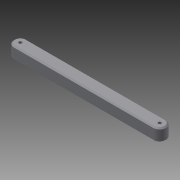
# Autodesk Inventor part: longerBar
Saved by Autodesk Inventor 2015 (Build 190159000, 159)
## iProperties
Created: 2015-04-09
Part Number: longerBar
Material: Generic
Document SubType Name: Modeling
Designer: WASHHSST
Density: 1 g/cm^3
Appearance: Default
Author: WASHHSST
Autodesk Inventor part; units mm, degrees
ref_plane "YZ Plane" through (0, 0, 0) normal (1, 0, 0) x (0, 1, 0)
ref_plane "XZ Plane" through (0, 0, 0) normal (0, 1, 0) x (-1, 0, 0)
sketch "Sketch1" plane through (0, 0, 0) normal (0, 1, 0) x (-1, 0, 0)
  line L0 (0, 0) -> (304.8, 0)
  line L1 (304.8, 0) -> (304.8, -25.4)
  line L2 (304.8, -25.4) -> (0, -25.4)
  line L3 (0, -25.4) -> (0, 0)
  dimension "d0" = 304.8
  dimension "d1" = 25.4
  constraints: 8 end point, 2 parallel, 1 horizontal, 1 perpendicular
  measures "d0" distance of L1.end L2.end
  measures "d1" distance of L0.end L1.end
extrude "Extrusion1" add sketch "Sketch1" along normal blind 25.4
hole "Hole1" at (-292.1, 25.4, -12.7) direction (0, -1, 0) diameter 6.35 end through all
ref_plane "Work Plane1" through (-152.4, 0, 0) normal (1, 0, 0) x (0, 0, -1)
mirror "Mirror1" about plane through (-152.4, 0, 0) normal (1, 0, 0) of "Hole1"
fillet "Fillet1" radius 12.7 4 edges at (-304.8, 12.7, -25.4) (-304.8, 12.7, 0) (0, 12.7, -25.4) (0, 12.7, 0)
chamfer "Chamfer1" distance 2.54 angle 45 8 edges at (-152.4, 25.4, 0) (-3.7197, 25.4, -21.6803) (-152.4, 25.4, -25.4) (-301.0803, 25.4, -21.6803) (-152.4, 0, 0) (-301.0803, 0, -21.6803) (-152.4, 0, -25.4) (-3.7197, 0, -21.6803)
body "Solid1"
